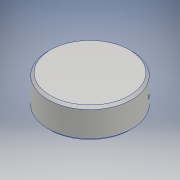
# Autodesk Inventor part: dummy_disc
Saved by Autodesk Inventor 2017 (Build 210142000, 142)
## iProperties
Created: 2017-09-28
Part Number: dummy_disc
Material: Aluminum 6061
Document SubType Name: Modeling
Designer: Thoma
Density: 2.7 g/cm^3
Appearance: Aluminum - Flat
Author: Thoma
Autodesk Inventor part; units mm, degrees
ref_plane "YZ Plane" through (0, 0, 0) normal (1, 0, 0) x (0, 1, 0)
ref_plane "XZ Plane" through (0, 0, 0) normal (0, 1, 0) x (-1, 0, 0)
ref_plane "XY Plane" through (0, 0, 0) normal (0, 0, 1) x (1, 0, 0)
sketch "Sketch1" plane through (0, 0, 0) normal (0, 0, 1) x (1, 0, 0)
  circle A0 centre (0, 0) radius 35
  dimension "d0" = 70
  constraints: 1 centre point, 1 coincident
  measures "d0" diameter of A0
extrude "Extrusion1" add sketch "Sketch1" along normal blind 25
chamfer "Chamfer1" distance 2 angle 45 2 edges at (-35, 0, 25) (-35, 0, 0)
sketch "Sketch2" plane through (0, 0, 25) normal (0, 0, 1) x (1, 0, 0)
  line L0 (0, 0) -> (0, 35) construction
  circle A0 centre (0, 0) radius 35 construction
  line L1 (0, 0) -> (35, 0) construction
  line L2 (0, 0) -> (27.4672, 21.6923) construction
  line L3 (0, 0) -> (35, 0) construction
  line L4 (0, 0) -> (18.9495, 29.4264) construction
  line L5 (0, 0) -> (35, 0) construction
  line L6 (0, 0) -> (-27.4672, 21.6923) construction
  line L7 (0, 0) -> (-18.9495, 29.4264) construction
  dimension "d6" = 38.3
  dimension "d7" = 57.22
  constraints: 16 end point, 4 point on circle, 2 equal length, 2 horizontal, 2 symmetric about line, 1 perpendicular
  measures "d6" angle of L3 L2
  measures "d7" angle of L5 L4
ref_plane "Work Plane1" through (27.4672, 21.6923, 25) normal (0.7847764, 0.619779, 0) x (-0.619779, 0.7847764, 0)
ref_plane "Work Plane2" through (18.9495, 29.4264, 25) normal (0.5414148, 0.8407556, 0) x (-0.8407556, 0.5414148, 0)
ref_plane "Work Plane3" through (-18.9495, 29.4264, 25) normal (-0.5414148, 0.8407556, 0) x (-0.8407556, -0.5414148, 0)
ref_plane "Work Plane4" through (-27.4672, 21.6923, 25) normal (-0.7847764, 0.619779, 0) x (-0.619779, -0.7847764, 0)
sketch "Sketch3" plane through (27.4672, 21.6923, 25) normal (0.7847764, 0.619779, 0) x (-0.619779, 0.7847764, 0)
  line L0 (-33, 0) -> (33, 0) projected
  point P0 (0, -25)
  point P1 (0, -14.5)
  dimension "d8" = 14.5
  measures "d8" distance from line of point (0, -14.5) L0
sketch "Sketch4" plane through (18.9495, 29.4264, 25) normal (0.5414148, 0.8407556, 0) x (-0.8407556, 0.5414148, 0)
  line L0 (-33, 0) -> (33, 0) projected
  point P0 (0, -25)
  point P1 (0, -14.5)
  dimension "d9" = 14.5
  measures "d9" distance from line of L0 point (0, -14.5)
sketch "Sketch5" plane through (-18.9495, 29.4264, 25) normal (-0.5414148, 0.8407556, 0) x (-0.8407556, -0.5414148, 0)
  line L0 (-33, 0) -> (33, 0) projected
  point P0 (0, -25)
  point P1 (0, -14.5)
  dimension "d10" = 14.5
  measures "d10" distance from line of L0 point (0, -14.5)
sketch "Sketch6" plane through (-27.4672, 21.6923, 25) normal (-0.7847764, 0.619779, 0) x (-0.619779, -0.7847764, 0)
  line L0 (-33, 0) -> (33, 0) projected
  point P0 (0, -25)
  point P1 (0, -14.5)
  dimension "d11" = 14.5
  measures "d11" distance from line of L0 point (0, -14.5)
hole "Hole1" at (-27.4672, 21.6923, 10.5) direction (0.7847764, -0.619779, 0) diameter 3 depth 8 tip angle 118
hole "Hole2" at (-18.9495, 29.4264, 10.5) direction (0.5414148, -0.8407556, 0) diameter 3 depth 8 tip angle 118
hole "Hole3" at (18.9495, 29.4264, 10.5) direction (-0.5414148, -0.8407556, 0) diameter 3 depth 8 tip angle 118
hole "Hole4" at (27.4672, 21.6923, 10.5) direction (-0.7847764, -0.619779, 0) diameter 3 depth 8 tip angle 118
thread "Thread1" size "M3x0.5" class "6H" standard "ANSI Metric M Profile" full length
thread "Thread2" size "M3x0.5" class "6H" standard "ANSI Metric M Profile" full length
thread "Thread3" size "M3x0.5" class "6H" standard "ANSI Metric M Profile" full length
thread "Thread4" size "M3x0.5" class "6H" standard "ANSI Metric M Profile" full length
body "Solid1"
